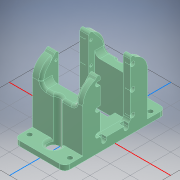
# Autodesk Inventor part: 000.005.002.001 - ОСНОВАНИЕ
Saved by Autodesk Inventor 2022 (Build 260153000, 153)
## iProperties
Created: 2022-11-19
Part Number: 000.005.002.001 - ОСНОВАНИЕ
Material: Пластик АБС
Document SubType Name: Modeling
Designer: Petrov Ivan
Density: 1.06 g/cm^3
Appearance: Гладкий — темный цвет морской волны
Mass: 84.8543 g
Surface Area: 271.699 cm^2
Volume: 80.0512 cm^3
Author: Petrov Ivan
Autodesk Inventor part; units mm, degrees
ref_plane "YZ Plane" through (0, 0, 0) normal (1, 0, 0) x (0, 1, 0)
ref_plane "XZ Plane" through (0, 0, 0) normal (0, 1, 0) x (-1, 0, 0)
ref_plane "XY Plane" through (0, 0, 0) normal (0, 0, 1) x (1, 0, 0)
sketch "Эскиз1" plane through (0, 0, 0) normal (0, 1, 0) x (-1, 0, 0)
  circle A0 centre (0, 0) radius 77.5
  circle A1 centre (20, 40) radius 2.5
  circle A2 centre (-20, 40) radius 2.5
  circle A3 centre (-20, -40) radius 2.5
  circle A4 centre (20, -40) radius 2.5
  line L0 (-25, 50) -> (25, 50)
  line L1 (25, 50) -> (25, -50)
  line L2 (25, -50) -> (-25, -50)
  line L3 (-25, -50) -> (-25, 50)
  line L4 (-25, 50) -> (25, -50) construction
  line L5 (25, 50) -> (-25, -50) construction
  dimension "d0" = 100
  dimension "d1" = 50
  constraints: 12 end point, 5 centre point, 2 midpoint, 2 parallel, 1 horizontal, 1 perpendicular, 1 point on line, 12 other
  measures "d0" distance of L0.end L1.end
  measures "d1" distance of L1.end L2.end
extrude "Выдавливание1" add sketch "Эскиз1" along normal blind 5 contours L0 L1 L2 L3
sketch "Эскиз2" plane through (-25, 0, -50) normal (-1, 0, 0) x (0, 0, 1)
  line L0 (35.5, 67.1) -> (35.5, 13.6) projected
  line L1 (35, 70.1) -> (38.5, 70.1) projected
  line L2 (35, 70.1) -> (29.9, 64.1) projected
  line L3 (29.9, 64.1) -> (29.9, 11) projected
  line L4 (29.9, 11) -> (35, 5) projected
  line L5 (35, 5) -> (65, 5) projected
  line L6 (65, 5) -> (70.1, 11) projected
  line L7 (70.1, 11) -> (70.1, 64.1) projected
  line L8 (70.1, 64.1) -> (65, 70.1) projected
  line L9 (61.5, 70.1) -> (65, 70.1) projected
  line L10 (64.5, 13.6) -> (64.5, 67.1) projected
  line L11 (38.5, 10.6) -> (61.5, 10.6) projected
  line L12 (61.5, 70.1) -> (38.5, 70.1) projected
  line L13 (70.1, 64.1) -> (82.1, 64.1)
  line L14 (82.1, 64.1) -> (82.1, 5)
  line L15 (0, 5) -> (100, 5) projected
  line L16 (100, 5) -> (0, 5) projected
  line L17 (50, 70.1) -> (50, -18.2992) construction
  line L18 (29.9, 64.1) -> (17.9, 64.1)
  line L19 (17.9, 64.1) -> (17.9, 5)
  line L20 (64.5, 67.1) -> (64.5, 70.1)
  line L21 (35.5, 67.1) -> (35.5, 70.1)
  arc A0 (38.5, 70.1) -> (35.5, 67.1) centre (38.5, 67.1) ccw projected
  arc A1 (64.5, 67.1) -> (61.5, 70.1) centre (61.5, 67.1) ccw projected
  arc A2 (61.5, 10.6) -> (64.5, 13.6) centre (61.5, 13.6) ccw projected
  arc A3 (35.5, 13.6) -> (38.5, 10.6) centre (38.5, 13.6) ccw projected
  circle A4 centre (39, 7.8) radius 1.35 projected
  circle A5 centre (32.7, 15.6) radius 1.35 projected
  circle A6 centre (32.7, 37.6) radius 1.35 projected
  circle A7 centre (32.7, 59.6) radius 1.35 projected
  circle A8 centre (61, 7.8) radius 1.35 projected
  circle A9 centre (67.3, 15.6) radius 1.35 projected
  circle A10 centre (67.3, 37.6) radius 1.35 projected
  circle A11 centre (67.3, 59.6) radius 1.35 projected
  point P0 (50, 0)
  point P1 (17.9, 5)
  dimension "d6" = 12
  constraints: 14 end point, 4 perpendicular, 4 point on line, 2 tangent, 1 midpoint, 1 vertical, 2 other
  measures "d6" distance between parallel lines of L7 L14
ref_plane "РабПлоскость1" through (-16.25, 5, -20.1) normal (-1, 0, 0) x (0, 0, 1)
extrude "Выдавливание2" add sketch "Эскиз2" against normal up to surface (8.75 mm away) contours L0 A3 L11 A2 L10 L20 L9 L8 L7 L6 L5 L4 L3 L2 L1 L21 | L3 L4 L15 L19 L18 | L13 L14 L15 L6 L7
fillet "Сопряжение1" radius 2 4 edges at (-20.625, 70.1, 15) (-20.625, 70.1, 14.5) (-20.625, 70.1, -14.5) (-20.625, 70.1, -15)
fillet "Сопряжение2" radius 17 2 edges at (-20.625, 64.1, 32.1) (-20.625, 64.1, -32.1)
sketch "Эскиз3" plane through (25, 0, 50) normal (1, 0, 0) x (0, 0, -1)
  circle A0 centre (32.7, 37.6) radius 1.35 projected
  circle A1 centre (39, 7.8) radius 1.35 projected
  circle A2 centre (67.3, 59.6) radius 1.35 projected
  circle A3 centre (67.3, 37.6) radius 1.35 projected
  circle A4 centre (67.3, 15.6) radius 1.35 projected
  circle A5 centre (61, 7.8) radius 1.35 projected
  circle A6 centre (32.7, 15.6) radius 1.35 projected
  circle A7 centre (32.7, 59.6) radius 1.35 projected
  line L0 (70.1, 64.1) -> (68.0239, 66.5425) projected
  arc A8 (68.0239, 66.5425) -> (64.5, 65.2472) centre (66.5, 65.2472) ccw projected
  line L1 (64.5, 65.2472) -> (64.5, 13.6) projected
  arc A9 (61.5, 10.6) -> (64.5, 13.6) centre (61.5, 13.6) ccw projected
  line L2 (61.5, 10.6) -> (38.5, 10.6) projected
  arc A10 (35.5, 13.6) -> (38.5, 10.6) centre (38.5, 13.6) ccw projected
  line L3 (35.5, 13.6) -> (35.5, 65.2472) projected
  arc A11 (35.5, 65.2472) -> (31.9761, 66.5425) centre (33.5, 65.2472) ccw projected
  line L4 (31.9761, 66.5425) -> (29.9, 64.1) projected
  line L5 (82.1, 5) -> (17.9, 5) projected
  arc A12 (82.1, 47.8519) -> (70.1, 64.1) centre (65.1, 47.8519) ccw projected
  arc A13 (29.9, 64.1) -> (17.9, 47.8519) centre (34.9, 47.8519) ccw projected
  line L6 (17.9, 47.8519) -> (17.9, 5) projected
  line L7 (82.1, 5) -> (82.1, 47.8519) projected
  point P0 (50, 0)
extrude "Выдавливание3" add sketch "Эскиз3" against normal blind 7
offset faces "Размер1" outward -0.5 faces at (-22.0833, 48.0315, 14.5) (-19.1667, 11.0019, 13) (-22.0833, 10.6, 3.8333) (-19.1667, 12.504, -14.2926) (-22.0833, 30.8157, -14.5) (20.3333, 10.7333, -12.3843) (22.6667, 48.0315, -14.5) (22.6667, 10.6, -3.8333) (20.3333, 10.8074, 12.596) (22.6667, 30.8157, 14.5)
sketch "Эскиз4" plane through (-25, 0, -50) normal (-1, 0, 0) x (0, 0, 1)
  circle A0 centre (32.7, 59.6) radius 1.35 projected
  circle A1 centre (32.7, 59.6) radius 2.3
  line L0 (35, 13.6) -> (35, 64.659) projected
  line L1 (32.7, 61.9) -> (35, 61.9)
  line L2 (32.7, 57.3) -> (35, 57.3)
  circle A2 centre (32.7, 37.6) radius 1.35 projected
  circle A3 centre (32.7, 37.6) radius 2.3
  line L3 (32.7, 39.9) -> (35, 39.9)
  line L4 (35, 35.3) -> (32.7, 35.3)
  circle A4 centre (32.7, 15.6) radius 1.35 projected
  circle A5 centre (32.7, 15.6) radius 2.3
  line L5 (32.7, 17.9) -> (35, 17.9)
  line L6 (32.7, 13.3) -> (35.0129, 13.3)
  circle A6 centre (39, 7.8) radius 1.35 projected
  circle A7 centre (39, 7.8) radius 2.3
  line L7 (61.5, 10.1) -> (38.5, 10.1) projected
  line L8 (36.7, 7.8) -> (36.7, 10.5983)
  arc A8 (35, 13.6) -> (38.5, 10.1) centre (38.5, 13.6) ccw projected
  line L9 (41.3, 7.8) -> (41.3, 10.1)
  line L10 (50, 0) -> (50, 3.8602) construction
  circle A9 centre (67.3, 59.6) radius 1.35
  circle A10 centre (67.3, 59.6) radius 2.3
  line L11 (65, 13.6) -> (65, 64.659)
  line L12 (67.3, 61.9) -> (65, 61.9)
  line L13 (67.3, 57.3) -> (65, 57.3)
  circle A11 centre (67.3, 37.6) radius 1.35
  circle A12 centre (67.3, 37.6) radius 2.3
  line L14 (67.3, 39.9) -> (65, 39.9)
  line L15 (65, 35.3) -> (67.3, 35.3)
  circle A13 centre (67.3, 15.6) radius 1.35
  circle A14 centre (67.3, 15.6) radius 2.3
  line L16 (67.3, 17.9) -> (65, 17.9)
  line L17 (67.3, 13.3) -> (64.9871, 13.3)
  circle A15 centre (61, 7.8) radius 1.35
  circle A16 centre (61, 7.8) radius 2.3
  line L18 (63.3, 7.8) -> (63.3, 10.5983)
  arc A17 (61.5, 10.1) -> (65, 13.6) centre (61.5, 13.6) ccw
  line L19 (58.7, 7.8) -> (58.7, 10.1)
  point P0 (35, 15.6)
  constraints: 36 end point, 27 symmetric about line, 22 point on circle, 13 centre point, 11 point on line, 10 tangent, 8 coincident, 4 perpendicular, 2 parallel, 2 vertical, 9 other
extrude "Выдавливание4" cut sketch "Эскиз4" against normal blind 5 contours A0 | A1 | A5 | A3 | A2 | A4 | A6 | A7 | L8 A8 L7 A7 | A7 L7 L9 | A17 L18 A16 L7 | A16 L19 L7 | A16 | A9 | A10 | A10 L11 L12 | L13 L11 A10 | L11 A14 L17 A17 | L11 L16 A14 | A14 | L11 A12 L15 | L11 L14 A12 | A12 | A11 | A13 | A15
mirror "Зеркальное отражение2" about plane through (0, 0, 0) normal (1, 0, 0) of "Выдавливание4"
sketch "Эскиз5" plane through (0, 5, 0) normal (0, 1, 0) x (1, 0, 0)
  circle A0 centre (0, 36) radius 6 projected
  circle A1 centre (0, -36) radius 6 projected
  point P0 (0, 0)
extrude "Выдавливание5" cut sketch "Эскиз5" against normal through all
fillet "Сопряжение4" radius 5 4 edges at (-25, 2.5, 50) (25, 2.5, 50) (25, 2.5, -50) (-25, 2.5, -50)
sketch "Эскиз6" plane through (0, 5, 0) normal (0, 1, 0) x (1, 0, 0)
  line L0 (-25, -32.1) -> (-16.25, -32.1) projected
  line L1 (18, -32.1) -> (18, 32.1) projected
  line L2 (18, -32.1) -> (18, -21.1)
  line L3 (18, -21.1) -> (-16.25, -21.1)
  line L4 (-16.25, -21.1) -> (-16.25, -32.1)
  circle A0 centre (0, -36) radius 6 projected
  line L5 (-16.25, -32.1) -> (-4.5596, -32.1)
  line L6 (4.5596, -32.1) -> (18, -32.1)
  point P0 (0, 0)
  dimension "d29" = 11
  constraints: 10 end point, 3 parallel, 2 horizontal, 2 perpendicular, 2 point on circle, 1 point on line
  measures "d29" distance of L2.end L2.start
extrude "Выдавливание6" add sketch "Эскиз6" along normal blind 38.818 contours L6 A0 L5 L4 L3 L1
mirror "Зеркальное отражение3" about plane through (0, 0, 0) normal (0, 0, 1) of "Выдавливание6"
sketch "Эскиз7" plane through (0, 5, 0) normal (0, 1, 0) x (1, 0, 0)
  line L0 (-16.25, -21.1) -> (3.75, -21.1)
  line L1 (3.75, -21.1) -> (3.75, -14.1)
  line L2 (3.75, -14.1) -> (-16.25, -14.1)
  line L3 (-16.25, -14.1) -> (-16.25, -21.1)
  line L4 (-16.25, -15) -> (-16.25, -18.5239) projected
  point P0 (0, 0)
  point P1 (-16.25, 308.1)
  dimension "d23" = 20
  dimension "d26" = 0
  constraints: 8 end point, 2 parallel, 1 perpendicular
  measures "d23" distance between parallel lines of L1 L3
  measures "d26" distance between parallel lines of L4 L3
extrude "Выдавливание7" cut sketch "Эскиз7" against normal through all
mirror "Зеркальное отражение4" about plane through (0, 0, 0) normal (0, 0, 1) of "Выдавливание7"
fillet "Сопряжение5" radius 4.75 4 edges at (-16.25, 43.818, 26.6) (18, 43.818, 26.6) (-16.25, 43.818, -26.6) (18, 43.818, -26.6)
fillet "Сопряжение6" radius 2.25 4 edges at (-2.0787, 5, 41.6284) (5.6284, 5, 33.9213) (-2.0787, 5, -41.6284) (5.6284, 5, -33.9213)
fillet "Сопряжение7" radius 2.5 18 edges at (16.3452, 44.965, 32.1) (17.9863, 48.208, 32.0963) (18, 58.2373, 28.559) (8.9048, 43.818, 32.1) (-14.5952, 44.965, 32.1) (-16.2363, 48.2081, 32.0963) (-16.25, 58.2373, 28.559) (-8.0298, 43.818, 32.1) (0, 43.818, 30) (16.3452, 44.965, -32.1) (17.9863, 48.2081, -32.0963) (18, 58.2373, -28.559) (8.9048, 43.818, -32.1) (0, 43.818, -30) (-14.5952, 44.965, -32.1) (-16.2363, 48.2081, -32.0963) (-16.25, 58.2373, -28.559) (-8.0298, 43.818, -32.1)
